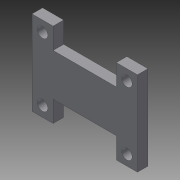
# Autodesk Inventor part: Stepper_Motor_Clamp
Saved by Autodesk Inventor 2015 (Build 190159000, 159)
## iProperties
Created: 2015-01-10
Part Number: Stepper_Motor_Clamp
Material: Generic
Document SubType Name: Modeling
Designer: Drew
Density: 1 g/cm^3
Appearance: Default
Author: Drew
Autodesk Inventor part; units mm, degrees
ref_plane "YZ Plane" through (0, 0, 0) normal (1, 0, 0) x (0, 1, 0)
ref_plane "XZ Plane" through (0, 0, 0) normal (0, 1, 0) x (-1, 0, 0)
ref_plane "XY Plane" through (0, 0, 0) normal (0, 0, 1) x (1, 0, 0)
sketch "Sketch1" plane through (0, 0, 0) normal (0, 0, 1) x (1, 0, 0)
  line L0 (-31.75, -25.4) -> (-31.75, 25.4)
  line L1 (31.75, 25.4) -> (31.75, -25.4)
  line L2 (31.75, -25.4) -> (-31.75, 25.4) construction
  line L3 (-31.75, -25.4) -> (31.75, 25.4) construction
  line L4 (-14.1411, 0) -> (14.1411, 0)
  line L5 (0, 15.3796) -> (0, -12.4523)
  line L6 (-19.05, 25.4) -> (-19.05, 12.7)
  line L7 (-19.05, 12.7) -> (19.05, 12.7)
  line L8 (19.05, 12.7) -> (19.05, 25.4)
  line L9 (-31.75, 25.4) -> (-19.05, 25.4)
  line L10 (19.05, 25.4) -> (31.75, 25.4)
  circle A0 centre (-25.4, 19.05) radius 3.175
  circle A1 centre (25.4, 19.05) radius 3.175
  circle A2 centre (-25.4, -19.05) radius 3.175
  circle A3 centre (25.4, -19.05) radius 3.175
  line L11 (19.05, -25.4) -> (19.05, -12.7)
  line L12 (19.05, -12.7) -> (-19.05, -12.7)
  line L13 (-19.05, -12.7) -> (-19.05, -25.4)
  line L14 (31.75, -25.4) -> (19.05, -25.4)
  line L15 (-19.05, -25.4) -> (-31.75, -25.4)
  point P0 (0, 0)
  point P1 (0, 0)
  point P2 (0, 0)
  point P3 (0, 0)
  dimension "d2" = 38.1
  dimension "d3" = 50.8
  dimension "d4" = 63.5
  dimension "d6" = 38.1
  dimension "d7" = 12.7
  dimension "d10" = 6.35
  dimension "d11" = 12.7
  dimension "d12" = 38.1
  dimension "d13" = 50.8
  constraints: 32 end point, 7 midpoint, 7 parallel, 7 perpendicular, 4 centre point, 3 horizontal, 3 symmetric about line, 3 vertical, 1 collinear, 1 point on line, 5 other
  measures "d2" distance of A2.centre A0.centre
  measures "d3" distance of A0.centre A1.centre
  measures "d4" distance of L1.end L0.start
  measures "d6" distance of L6.end L7.end
  measures "d7" distance of L6.start L6.end
  measures "d10" diameter of A1
  measures "d11" distance of L11.start L11.end
  measures "d12" distance of L11.end L12.end
  measures "d13" distance of L0.start L0.end
extrude "Extrusion1" add sketch "Sketch1" along normal blind 6.35
equation "\"d11\" = d7"
equation "\"d12\" = d6"
body "Solid1"
